LACK Controller Wire Holder (Autodesk Fusion 360 design; units mm, degrees)
Autodesk Fusion 360 part; units mm, degrees
note: some values were not read from the file. Set by a fixed rule: which sketch regions a step uses.
sketch "Sketch1" plane through (0, 0, 0) normal (0, 0, 1) x (1, 0, 0)
  line L0 (-12.5, 10) -> (12.5, 10)
  line L1 (12.5, 10) -> (12.5, -10)
  line L2 (12.5, -10) -> (-12.5, -10)
  line L3 (-12.5, -10) -> (-12.5, 10)
  dimension "d1" = 25
  dimension "d2" = 20
  dimension "d3" = 10
  dimension "d4" = 12.5
  constraint horizontal L0
  constraint vertical L1
  constraint horizontal L2
  constraint vertical L3
  measures "d1" distance of L1 L3
  measures "d2" distance of L0 L2
  measures "d3" distance of origin L2
  measures "d4" distance of origin L3
extrude "Extrude1" add sketch "Sketch1" along normal blind 2 makes body 1
sketch "Sketch2" plane through (0, 0, 2) normal (0, 0, 1) x (-1, 0, 0)
  line L0 (12.5, 10) -> (-12.5, 10)
  line L1 (-12.5, 10) -> (-12.5, -10)
  line L2 (-12.5, -10) -> (12.5, -10)
  line L3 (12.5, -10) -> (12.5, 10)
  line L4 (12.5, -10) -> (14.5, -10)
  line L5 (14.5, -10) -> (14.5, 10)
  line L6 (14.5, 10) -> (12.5, 10)
  line L7 (12.5, 10) -> (12.5, -10)
  dimension "d7" = 2
  constraint horizontal L4
  constraint vertical L5
  constraint horizontal L6
  constraint vertical L7
  constraint coincident L2.end L3.start
  constraint horizontal L0.start L5.end
  measures "d7" distance of L5 L7
extrude "Extrude2" add sketch "Sketch2" against normal blind 52 contours L3 L4 L5 L6 L7 bodies 1
sketch "Sketch3" plane through (0, 0, -50) normal (0, 0, -1) x (1, 0, 0)
  line L0 (-12.5, -10) -> (-12.5, 10)
  line L1 (-12.5, 10) -> (-14.5, 10)
  line L2 (-14.5, 10) -> (-14.5, -10)
  line L3 (-14.5, -10) -> (-12.5, -10)
  line L4 (-14.5, 10) -> (12.5, 10)
  line L5 (12.5, 10) -> (12.5, -10)
  line L6 (12.5, -10) -> (-14.5, -10)
  line L7 (-14.5, -10) -> (-14.5, 10)
  dimension "d10" = 27
  constraint horizontal L4
  constraint vertical L5
  constraint horizontal L6
  constraint vertical L7
  constraint horizontal L2.end L5.end
  constraint horizontal L1.end L2.start
  constraint vertical L1.end L2.end
  measures "d10" distance of L5 L7
extrude "Extrude3" add sketch "Sketch3" along normal blind 2 separate body makes body 2
ref_plane "WorkPlane1" through (-9, 0, 1) normal (1, 0, 0) x (0, 1, 0)
sketch "Sketch5" plane through (-9, 0, 0) normal (1, 0, 0) x (0, 1, 0)
  circle A0 centre (-0.375, 5.5) radius 2.75
  circle A1 centre (0.375, 5.5) radius 2.75
  circle A2 centre (-0.375, 5.5) radius 1.5
  circle A3 centre (0.375, 5.5) radius 1.5
  line L0 (-10, 2) -> (10, 2)
  line L1 (-0.375, 5.5) -> (-0.375, 2)
  line L2 (0.375, 5.5) -> (0.375, 2)
  line L3 (-0.375, 5.5) -> (-0.375, 16.5)
  line L4 (-0.375, 16.5) -> (0.375, 16.5)
  line L5 (0.375, 16.5) -> (0.375, 5.5)
  line L6 (-10, 4) -> (10, 4)
  line L7 (-10, 2) -> (-10, 4)
  line L8 (10, 2) -> (10, 4)
  point P0 (-10, 2)
  point P1 (10, 2)
  dimension "d14" = 5.5
  dimension "d15" = 5.5
  dimension "d16" = 5.5
  dimension "d17" = 0.75
  dimension "d18" = 0.375
  dimension "d19" = 3
  dimension "d20" = 3
  dimension "d21" = 2
  dimension "d42" = 1.5
  dimension "d43" = 20
  dimension "d44" = 10
  constraint horizontal A0.centre A1.centre
  constraint concentric A0 A2
  constraint concentric A1 A3
  constraint horizontal L0
  constraint coincident A0.centre A2.centre
  constraint coincident L0 L1.end
  constraint perpendicular L0 L1
  constraint coincident A1.centre A3.centre
  constraint coincident L0 L2.end
  constraint perpendicular L0 L2
  constraint parallel L2 L3
  constraint perpendicular L3 L4
  constraint perpendicular L4 L5
  constraint vertical P0 L0.start
  constraint vertical P1 L0.end
  constraint horizontal L6
  constraint coincident P0 L0.start
  measures "d14" diameter of A0
  measures "d15" diameter of A1
  measures "d16" vertical distance of origin A0.centre
  measures "d17" distance of A0.centre A1.centre
  measures "d18" horizontal distance of origin A1.centre
  measures "d19" diameter of A2
  measures "d20" diameter of A3
  measures "d21" distance of origin L0
  measures "d42" distance of A1.centre L6
  measures "d43" distance of L6.start L6.end
  measures "d44" horizontal distance of origin L6.end
extrude "Extrude6" add 1 faces at (4.1667, 3.3333, -50) along direction (0, 0, 1) blind 0.25 on bodies 2 bodies 1 2
extrude "Extrude7" cut 1 faces at (-5.5, -3.3333, -52) along direction (0, 0, 1) blind 0.25 on bodies 1 bodies 1
extrude "Extrude8" add sketch "Sketch5" along normal mid plane 3 contours A0 A3 L5 L6 | A0 A1 L5 L6 | A0 A1 L2 L6 | A0 L2 L6 | A0 A1 L2 | A0 A1 L1 L2 L6 | A1 L0 L2 L6 L8 | A0 A1 L3 L6 | A1 A2 L3 L6 | A0 A1 L0 L1 L2 | A0 A1 L1 | A1 L1 L6 | A0 A1 L1 L6 | A0 L0 L1 L6 L7 bodies 1
fillet "Fillet4" radius 0.5 2 edges at (-9, -0.375, 8.25) (-9, 0.375, 8.25) on bodies 1
fillet "Fillet4" radius 50 2 edges at (-9, -2.6799, 4) (-9, 2.6799, 4) on bodies 1
fillet "Fillet5" radius 2 2 edges at (-7.5, 0, 2) (-10.5, 0, 2) on bodies 1
fillet "Fillet6" radius 2 2 edges at (-9, -10, 4) (-9, 10, 4) on bodies 1
equation "d4 = 2.5 / 2 * 1 cm"
equation "d18 = ( 0.75 / 2 ) * 1 mm"
